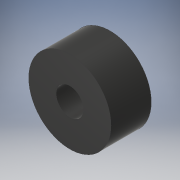
# Autodesk Inventor part: CLB_050_ScissorSliderSpacer
Saved by Autodesk Inventor 2018.3 (Build 223284000, 284)
## iProperties
Created: 2020-02-14
Part Number: CLB_050_ScissorSliderSpacer
Material: Acetal Resin, Black
Document SubType Name: Modeling
Designer: 22perngrac
Density: 1.425 g/cm^3
Appearance: Smooth - Black
Author: 22perngrac
Autodesk Inventor part; units mm, degrees
ref_plane "YZ Plane" through (0, 0, 0) normal (1, 0, 0) x (0, 1, 0)
ref_plane "XZ Plane" through (0, 0, 0) normal (0, 1, 0) x (-1, 0, 0)
ref_plane "XY Plane" through (0, 0, 0) normal (0, 0, 1) x (1, 0, 0)
sketch "Sketch2" plane through (0, 0, 0) normal (0, 0, 1) x (1, 0, 0)
  circle A0 centre (0, 0) radius 9.525
  dimension "d16" = 19.05
  constraints: 1 centre point, 1 coincident
  measures "d16" diameter of A0
extrude "Extrusion2" add sketch "Sketch2" along normal blind 9.3218
sketch "Sketch3" plane through (0, 0, 9.3218) normal (0, 0, 1) x (1, 0, 0)
  point P0 (0, 0)
hole "Hole1" at (0, 0, 9.3218) direction (0, 0, -1) diameter 6.35 end through all
body "Solid2"
